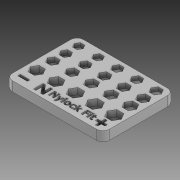
# Autodesk Inventor part: Standard Test Print
Saved by Autodesk Inventor 2022 (Build 260153000, 153)
## iProperties
Created: 2022-01-18
Part Number: Standard Test Print
Material: ABS Plastic
Document SubType Name: Modeling
Density: 1.06 g/cm^3
Appearance: Smooth - Medium Gray
Autodesk Inventor part; units mm, degrees
ref_plane "YZ Plane" through (0, 0, 0) normal (1, 0, 0) x (0, 1, 0)
ref_plane "XZ Plane" through (0, 0, 0) normal (0, 1, 0) x (-1, 0, 0)
ref_plane "XY Plane" through (0, 0, 0) normal (0, 0, 1) x (1, 0, 0)
sketch "Sketch1" plane through (0, 0, 0) normal (0, 1, 0) x (-1, 0, 0)
  line L0 (42.8625, 28.1781) -> (33.3375, 28.1781)
  line L1 (33.3375, 28.1781) -> (33.3375, 25.7969)
  line L2 (33.3375, 25.7969) -> (42.8625, 25.7969)
  line L3 (42.8625, 25.7969) -> (42.8625, 28.1781)
  line L4 (42.8625, 28.1781) -> (33.3375, 25.7969) construction
  line L5 (33.3375, 28.1781) -> (42.8625, 25.7969) construction
  line L6 (-33.3375, 28.1781) -> (-42.8625, 28.1781)
  line L7 (-42.8625, 28.1781) -> (-42.8625, 25.7969)
  line L8 (-42.8625, 25.7969) -> (-33.3375, 25.7969)
  line L9 (-33.3375, 25.7969) -> (-33.3375, 28.1781)
  line L10 (-33.3375, 28.1781) -> (-42.8625, 25.7969) construction
  line L11 (-42.8625, 28.1781) -> (-33.3375, 25.7969) construction
  line L12 (23.8125, 31.75) -> (23.8125, 22.225)
  line L13 (23.8125, 22.225) -> (21.4312, 22.225)
  line L14 (21.4312, 22.225) -> (16.6687, 28.0052)
  line L15 (16.6687, 28.0052) -> (16.6687, 22.225)
  line L16 (16.6687, 22.225) -> (14.2875, 22.225)
  line L17 (14.2875, 22.225) -> (14.2875, 31.75)
  line L18 (14.2875, 31.75) -> (16.6687, 31.75)
  line L19 (16.6687, 31.75) -> (21.4312, 25.9698)
  line L20 (21.4312, 25.9698) -> (21.4312, 31.75)
  line L21 (21.4312, 31.75) -> (23.8125, 31.75)
  line L22 (19.05, 28.8599) -> (19.05, 25.1151) construction
  line L23 (47.625, -34.925) -> (-47.625, -34.925)
  line L24 (-47.625, -34.925) -> (-47.625, 34.925)
  line L25 (-47.625, 34.925) -> (47.625, 34.925)
  line L26 (47.625, 34.925) -> (47.625, -34.925)
  line L27 (47.625, -34.925) -> (-47.625, 34.925) construction
  line L28 (-47.625, -34.925) -> (47.625, 34.925) construction
  line L29 (-39.2906, 22.225) -> (-36.9094, 22.225)
  line L30 (-36.9094, 22.225) -> (-36.9094, 31.75)
  line L31 (-36.9094, 31.75) -> (-39.2906, 31.75)
  line L32 (-39.2906, 31.75) -> (-39.2906, 22.225)
  line L33 (-39.2906, 22.225) -> (-36.9094, 31.75) construction
  line L34 (-36.9094, 22.225) -> (-39.2906, 31.75) construction
  line L35 (35.8086, -30.9562) -> (33.5173, -26.9875) construction
  line L36 (33.5173, -26.9875) -> (35.8086, -23.0187) construction
  line L37 (35.8086, -23.0187) -> (40.3914, -23.0187) construction
  line L38 (40.3914, -23.0187) -> (42.6827, -26.9875) construction
  line L39 (42.6827, -26.9875) -> (40.3914, -30.9563) construction
  line L40 (40.3914, -30.9563) -> (35.8086, -30.9562) construction
  line L41 (35.5795, -18.6531) -> (33.059, -14.2875) construction
  line L42 (33.059, -14.2875) -> (35.5795, -9.9219) construction
  line L43 (35.5795, -9.9219) -> (40.6205, -9.9219) construction
  line L44 (40.6205, -9.9219) -> (43.141, -14.2875) construction
  line L45 (43.141, -14.2875) -> (40.6205, -18.6531) construction
  line L46 (40.6205, -18.6531) -> (35.5795, -18.6531) construction
  line L47 (35.3504, -6.35) -> (32.6007, -1.5875) construction
  line L48 (32.6007, -1.5875) -> (35.3504, 3.175) construction
  line L49 (35.3504, 3.175) -> (40.8496, 3.175) construction
  line L50 (40.8496, 3.175) -> (43.5993, -1.5875) construction
  line L51 (43.5993, -1.5875) -> (40.8496, -6.35) construction
  line L52 (40.8496, -6.35) -> (35.3504, -6.35) construction
  line L53 (34.8921, 8.7312) -> (31.6842, 14.2875) construction
  line L54 (31.6842, 14.2875) -> (34.8921, 19.8437) construction
  line L55 (34.8921, 19.8437) -> (41.3079, 19.8438) construction
  line L56 (41.3079, 19.8438) -> (44.5158, 14.2875) construction
  line L57 (44.5158, 14.2875) -> (41.3079, 8.7312) construction
  line L58 (41.3079, 8.7312) -> (34.8921, 8.7312) construction
  line L59 (15.8421, 8.7312) -> (12.6342, 14.2875)
  line L60 (12.6342, 14.2875) -> (15.8421, 19.8437)
  line L61 (22.2579, 8.7312) -> (15.8421, 8.7312)
  line L62 (15.8421, 19.8437) -> (22.2579, 19.8438)
  line L63 (25.4658, 14.2875) -> (22.2579, 8.7312)
  line L64 (22.2579, 19.8438) -> (25.4658, 14.2875)
  line L65 (16.3004, 3.175) -> (21.7996, 3.175)
  line L66 (21.7996, 3.175) -> (24.5493, -1.5875)
  line L67 (24.5493, -1.5875) -> (21.7996, -6.35)
  line L68 (21.7996, -6.35) -> (16.3004, -6.35)
  line L69 (21.5705, -9.9219) -> (24.091, -14.2875)
  line L70 (16.5295, -18.6531) -> (14.009, -14.2875)
  line L71 (24.091, -14.2875) -> (21.5705, -18.6531)
  line L72 (21.5705, -18.6531) -> (16.5295, -18.6531)
  line L73 (16.7586, -23.0187) -> (21.3414, -23.0187)
  line L74 (14.4673, -26.9875) -> (16.7586, -23.0187)
  line L75 (16.7586, -30.9562) -> (14.4673, -26.9875)
  line L76 (21.3414, -30.9563) -> (16.7586, -30.9562)
  line L77 (21.3414, -23.0187) -> (23.6327, -26.9875)
  line L78 (23.6327, -26.9875) -> (21.3414, -30.9563)
  line L79 (16.5295, -9.9219) -> (21.5705, -9.9219)
  line L80 (13.5507, -1.5875) -> (16.3004, 3.175)
  line L81 (16.3004, -6.35) -> (13.5507, -1.5875)
  line L82 (14.009, -14.2875) -> (16.5295, -9.9219)
  line L83 (-3.2079, 8.7312) -> (-6.4158, 14.2875) construction
  line L84 (-6.4158, 14.2875) -> (-3.2079, 19.8437) construction
  line L85 (3.2079, 8.7312) -> (-3.2079, 8.7312) construction
  line L86 (-3.2079, 19.8437) -> (3.2079, 19.8438) construction
  line L87 (6.4158, 14.2875) -> (3.2079, 8.7312) construction
  line L88 (3.2079, 19.8438) -> (6.4158, 14.2875) construction
  line L89 (-2.7496, 3.175) -> (2.7496, 3.175) construction
  line L90 (2.7496, 3.175) -> (5.4993, -1.5875) construction
  line L91 (5.4993, -1.5875) -> (2.7496, -6.35) construction
  line L92 (2.7496, -6.35) -> (-2.7496, -6.35) construction
  line L93 (2.5205, -9.9219) -> (5.041, -14.2875) construction
  line L94 (-2.5205, -18.6531) -> (-5.041, -14.2875) construction
  line L95 (5.041, -14.2875) -> (2.5205, -18.6531) construction
  line L96 (2.5205, -18.6531) -> (-2.5205, -18.6531) construction
  line L97 (-2.2914, -23.0187) -> (2.2914, -23.0187) construction
  line L98 (-4.5827, -26.9875) -> (-2.2914, -23.0187) construction
  line L99 (-2.2914, -30.9562) -> (-4.5827, -26.9875) construction
  line L100 (2.2914, -30.9563) -> (-2.2914, -30.9562) construction
  line L101 (2.2914, -23.0187) -> (4.5827, -26.9875) construction
  line L102 (4.5827, -26.9875) -> (2.2914, -30.9563) construction
  line L103 (-2.5205, -9.9219) -> (2.5205, -9.9219) construction
  line L104 (-5.4993, -1.5875) -> (-2.7496, 3.175) construction
  line L105 (-2.7496, -6.35) -> (-5.4993, -1.5875) construction
  line L106 (-5.041, -14.2875) -> (-2.5205, -9.9219) construction
  line L107 (-22.2579, 8.7312) -> (-25.4658, 14.2875) construction
  line L108 (-25.4658, 14.2875) -> (-22.2579, 19.8437) construction
  line L109 (-15.8421, 8.7312) -> (-22.2579, 8.7312) construction
  line L110 (-22.2579, 19.8437) -> (-15.8421, 19.8438) construction
  line L111 (-12.6342, 14.2875) -> (-15.8421, 8.7312) construction
  line L112 (-15.8421, 19.8438) -> (-12.6342, 14.2875) construction
  line L113 (-21.7996, 3.175) -> (-16.3004, 3.175) construction
  line L114 (-16.3004, 3.175) -> (-13.5507, -1.5875) construction
  line L115 (-13.5507, -1.5875) -> (-16.3004, -6.35) construction
  line L116 (-16.3004, -6.35) -> (-21.7996, -6.35) construction
  line L117 (-16.5295, -9.9219) -> (-14.009, -14.2875) construction
  line L118 (-21.5705, -18.6531) -> (-24.091, -14.2875) construction
  line L119 (-14.009, -14.2875) -> (-16.5295, -18.6531) construction
  line L120 (-16.5295, -18.6531) -> (-21.5705, -18.6531) construction
  line L121 (-21.3414, -23.0187) -> (-16.7586, -23.0187) construction
  line L122 (-23.6327, -26.9875) -> (-21.3414, -23.0187) construction
  line L123 (-21.3414, -30.9562) -> (-23.6327, -26.9875) construction
  line L124 (-16.7586, -30.9563) -> (-21.3414, -30.9562) construction
  line L125 (-16.7586, -23.0187) -> (-14.4673, -26.9875) construction
  line L126 (-14.4673, -26.9875) -> (-16.7586, -30.9563) construction
  line L127 (-21.5705, -9.9219) -> (-16.5295, -9.9219) construction
  line L128 (-24.5493, -1.5875) -> (-21.7996, 3.175) construction
  line L129 (-21.7996, -6.35) -> (-24.5493, -1.5875) construction
  line L130 (-24.091, -14.2875) -> (-21.5705, -9.9219) construction
  line L131 (-41.3079, 8.7312) -> (-44.5158, 14.2875) construction
  line L132 (-44.5158, 14.2875) -> (-41.3079, 19.8437) construction
  line L133 (-34.8921, 8.7312) -> (-41.3079, 8.7312) construction
  line L134 (-41.3079, 19.8437) -> (-34.8921, 19.8438) construction
  line L135 (-31.6842, 14.2875) -> (-34.8921, 8.7312) construction
  line L136 (-34.8921, 19.8438) -> (-31.6842, 14.2875) construction
  line L137 (-40.8496, 3.175) -> (-35.3504, 3.175) construction
  line L138 (-35.3504, 3.175) -> (-32.6007, -1.5875) construction
  line L139 (-32.6007, -1.5875) -> (-35.3504, -6.35) construction
  line L140 (-35.3504, -6.35) -> (-40.8496, -6.35) construction
  line L141 (-35.5795, -9.9219) -> (-33.059, -14.2875) construction
  line L142 (-40.6205, -18.6531) -> (-43.141, -14.2875) construction
  line L143 (-33.059, -14.2875) -> (-35.5795, -18.6531) construction
  line L144 (-35.5795, -18.6531) -> (-40.6205, -18.6531) construction
  line L145 (-40.3914, -23.0187) -> (-35.8086, -23.0187) construction
  line L146 (-42.6827, -26.9875) -> (-40.3914, -23.0187) construction
  line L147 (-40.3914, -30.9562) -> (-42.6827, -26.9875) construction
  line L148 (-35.8086, -30.9563) -> (-40.3914, -30.9562) construction
  line L149 (-35.8086, -23.0187) -> (-33.5173, -26.9875) construction
  line L150 (-33.5173, -26.9875) -> (-35.8086, -30.9563) construction
  line L151 (-40.6205, -9.9219) -> (-35.5795, -9.9219) construction
  line L152 (-43.5993, -1.5875) -> (-40.8496, 3.175) construction
  line L153 (-40.8496, -6.35) -> (-43.5993, -1.5875) construction
  line L154 (-43.141, -14.2875) -> (-40.6205, -9.9219) construction
  line L155 (33.6639, -26.9875) -> (35.882, -30.8293)
  line L156 (35.882, -30.8293) -> (40.318, -30.8292)
  line L157 (40.318, -30.8292) -> (42.5361, -26.9875)
  line L158 (42.5361, -26.9875) -> (40.318, -23.1457)
  line L159 (40.318, -23.1457) -> (35.882, -23.1458)
  line L160 (35.882, -23.1458) -> (33.6639, -26.9875)
  line L161 (35.6528, -18.5261) -> (33.2057, -14.2875)
  line L162 (33.2057, -14.2875) -> (35.6528, -10.0489)
  line L163 (35.6528, -10.0489) -> (40.5472, -10.0489)
  line L164 (40.5472, -10.0489) -> (42.9943, -14.2875)
  line L165 (42.9943, -14.2875) -> (40.5472, -18.5261)
  line L166 (40.5472, -18.5261) -> (35.6528, -18.5261)
  line L167 (35.4237, -6.223) -> (32.7474, -1.5875)
  line L168 (32.7474, -1.5875) -> (35.4237, 3.048)
  line L169 (35.4237, 3.048) -> (40.7763, 3.048)
  line L170 (40.7763, 3.048) -> (43.4526, -1.5875)
  line L171 (43.4526, -1.5875) -> (40.7763, -6.223)
  line L172 (40.7763, -6.223) -> (35.4237, -6.223)
  line L173 (34.9654, 8.8583) -> (31.8308, 14.2875)
  line L174 (31.8308, 14.2875) -> (34.9654, 19.7167)
  line L175 (34.9654, 19.7167) -> (41.2346, 19.7167)
  line L176 (41.2346, 19.7167) -> (44.3692, 14.2875)
  line L177 (44.3692, 14.2875) -> (41.2346, 8.8583)
  line L178 (41.2346, 8.8583) -> (34.9654, 8.8583)
  line L179 (4.876, -26.9875) -> (2.438, -22.7647)
  line L180 (2.438, -22.7647) -> (-2.438, -22.7647)
  line L181 (-2.438, -22.7647) -> (-4.876, -26.9875)
  line L182 (-4.876, -26.9875) -> (-2.438, -31.2102)
  line L183 (-2.438, -31.2102) -> (2.438, -31.2102)
  line L184 (2.438, -31.2102) -> (4.876, -26.9875)
  line L185 (2.6671, -18.9071) -> (5.3343, -14.2875)
  line L186 (5.3343, -14.2875) -> (2.6671, -9.6679)
  line L187 (2.6671, -9.6679) -> (-2.6671, -9.6679)
  line L188 (-2.6671, -9.6679) -> (-5.3343, -14.2875)
  line L189 (-5.3343, -14.2875) -> (-2.6671, -18.9071)
  line L190 (-2.6671, -18.9071) -> (2.6671, -18.9071)
  line L191 (5.7926, -1.5875) -> (2.8963, 3.429)
  line L192 (2.8963, 3.429) -> (-2.8963, 3.429)
  line L193 (-2.8963, 3.429) -> (-5.7926, -1.5875)
  line L194 (-5.7926, -1.5875) -> (-2.8963, -6.604)
  line L195 (-2.8963, -6.604) -> (2.8963, -6.604)
  line L196 (2.8963, -6.604) -> (5.7926, -1.5875)
  line L197 (3.3545, 8.4773) -> (6.7091, 14.2875)
  line L198 (6.7091, 14.2875) -> (3.3545, 20.0977)
  line L199 (3.3545, 20.0977) -> (-3.3545, 20.0977)
  line L200 (-3.3545, 20.0977) -> (-6.7091, 14.2875)
  line L201 (-6.7091, 14.2875) -> (-3.3545, 8.4773)
  line L202 (-3.3545, 8.4773) -> (3.3545, 8.4773)
  line L203 (-12.1943, 14.2875) -> (-15.6221, 20.2247)
  line L204 (-15.6221, 20.2247) -> (-22.4779, 20.2247)
  line L205 (-22.4779, 20.2247) -> (-25.9057, 14.2875)
  line L206 (-25.9057, 14.2875) -> (-22.4779, 8.3502)
  line L207 (-22.4779, 8.3502) -> (-15.6221, 8.3502)
  line L208 (-15.6221, 8.3502) -> (-12.1943, 14.2875)
  line L209 (-13.1108, -1.5875) -> (-16.0804, 3.556)
  line L210 (-16.0804, 3.556) -> (-22.0196, 3.556)
  line L211 (-22.0196, 3.556) -> (-24.9892, -1.5875)
  line L212 (-24.9892, -1.5875) -> (-22.0196, -6.731)
  line L213 (-22.0196, -6.731) -> (-16.0804, -6.731)
  line L214 (-16.0804, -6.731) -> (-13.1108, -1.5875)
  line L215 (-13.5691, -14.2875) -> (-16.3095, -9.5409)
  line L216 (-16.3095, -9.5409) -> (-21.7905, -9.5409)
  line L217 (-21.7905, -9.5409) -> (-24.5309, -14.2875)
  line L218 (-24.5309, -14.2875) -> (-21.7905, -19.0341)
  line L219 (-21.7905, -19.0341) -> (-16.3095, -19.0341)
  line L220 (-16.3095, -19.0341) -> (-13.5691, -14.2875)
  line L221 (-14.0273, -26.9875) -> (-16.5387, -22.6378)
  line L222 (-16.5387, -22.6378) -> (-21.5613, -22.6378)
  line L223 (-21.5613, -22.6378) -> (-24.0727, -26.9875)
  line L224 (-24.0727, -26.9875) -> (-21.5613, -31.3372)
  line L225 (-21.5613, -31.3372) -> (-16.5387, -31.3372)
  line L226 (-16.5387, -31.3372) -> (-14.0273, -26.9875)
  line L227 (-35.5153, -31.4642) -> (-32.9307, -26.9875)
  line L228 (-32.9307, -26.9875) -> (-35.5153, -22.5108)
  line L229 (-35.5153, -22.5108) -> (-40.6847, -22.5108)
  line L230 (-40.6847, -22.5108) -> (-43.2693, -26.9875)
  line L231 (-43.2693, -26.9875) -> (-40.6847, -31.4642)
  line L232 (-40.6847, -31.4642) -> (-35.5153, -31.4642)
  line L233 (-32.4724, -14.2875) -> (-35.2862, -9.4139)
  line L234 (-35.2862, -9.4139) -> (-40.9138, -9.4139)
  line L235 (-40.9138, -9.4139) -> (-43.7276, -14.2875)
  line L236 (-43.7276, -14.2875) -> (-40.9138, -19.1611)
  line L237 (-40.9138, -19.1611) -> (-35.2862, -19.1611)
  line L238 (-35.2862, -19.1611) -> (-32.4724, -14.2875)
  line L239 (-32.0142, -1.5875) -> (-35.0571, 3.683)
  line L240 (-35.0571, 3.683) -> (-41.1429, 3.683)
  line L241 (-41.1429, 3.683) -> (-44.1858, -1.5875)
  line L242 (-44.1858, -1.5875) -> (-41.1429, -6.858)
  line L243 (-41.1429, -6.858) -> (-35.0571, -6.858)
  line L244 (-35.0571, -6.858) -> (-32.0142, -1.5875)
  line L245 (-34.5988, 8.2233) -> (-31.0976, 14.2875)
  line L246 (-31.0976, 14.2875) -> (-34.5988, 20.3518)
  line L247 (-34.5988, 20.3518) -> (-41.6012, 20.3518)
  line L248 (-41.6012, 20.3518) -> (-45.1024, 14.2875)
  line L249 (-45.1024, 14.2875) -> (-41.6012, 8.2233)
  line L250 (-41.6012, 8.2233) -> (-34.5988, 8.2233)
  line L251 (16.0071, 23.8369) -> (-35.0571, 23.8369) construction
  line L252 (-35.0571, 23.8369) -> (-35.0571, 30.1381) construction
  line L253 (-35.0571, 30.1381) -> (16.0071, 30.1381) construction
  line L254 (16.0071, 30.1381) -> (16.0071, 23.8369) construction
  line L255 (6.1493, 29.4292) -> (7.6828, 29.4292)
  line L256 (7.6828, 29.4292) -> (10.1322, 25.0038)
  line L257 (10.1322, 25.0038) -> (10.1322, 29.4292)
  line L258 (10.1322, 29.4292) -> (11.5885, 29.4292)
  line L259 (11.5885, 29.4292) -> (11.5885, 23.0792)
  line L260 (11.5885, 23.0792) -> (9.6331, 23.0792)
  line L261 (9.6331, 23.0792) -> (7.6056, 26.7173)
  line L262 (7.6056, 26.7173) -> (7.6056, 23.0792)
  line L263 (7.6056, 23.0792) -> (6.1493, 23.0792)
  line L264 (6.1493, 23.0792) -> (6.1493, 29.4292)
  line L265 (0.4786, 24.6384) -> (2.892, 31.184)
  line L266 (2.892, 31.184) -> (4.4975, 31.184)
  line L267 (4.4975, 31.184) -> (3.7719, 29.3109)
  line L268 (3.7719, 29.3109) -> (5.5267, 24.6384)
  line L269 (5.5267, 24.6384) -> (3.9623, 24.6384)
  line L270 (3.9623, 24.6384) -> (2.9537, 27.6436)
  line L271 (2.9537, 27.6436) -> (2.012, 24.6384)
  line L272 (2.012, 24.6384) -> (0.4786, 24.6384)
  line L273 (-1.5746, 29.4292) -> (-0.0823, 29.4292)
  line L274 (-0.0823, 29.4292) -> (-0.0823, 22.7962)
  line L275 (-0.0823, 22.7962) -> (-1.5746, 22.7962)
  line L276 (-1.5746, 22.7962) -> (-1.5746, 29.4292)
  spline S0 degree 2 poles (-7.3123, 27.0364) (-7.3123, 28.2199) (-6.0207, 29.5784) (-4.8423, 29.5784) knots 0 0 0 1 2 2 2
  spline S1 degree 2 poles (-4.8423, 29.5784) (-3.669, 29.5784) (-2.3671, 28.2199) (-2.3671, 27.0364) knots 0 0 0 1 2 2 2
  spline S2 degree 2 poles (-2.3671, 27.0364) (-2.3671, 25.8425) (-3.669, 24.4892) (-4.8423, 24.4892) knots 0 0 0 1 2 2 2
  spline S3 degree 2 poles (-4.8423, 24.4892) (-6.0155, 24.4892) (-7.3123, 25.8477) (-7.3123, 27.0364) knots 0 0 0 1 2 2 2
  spline S4 degree 2 poles (-5.784, 27.0467) (-5.784, 26.6196) (-5.645, 26.0484) (-5.5215, 25.8786) knots 0 0 0 1 2 2 2
  spline S5 degree 2 poles (-5.5215, 25.8786) (-5.3877, 25.6985) (-5.0532, 25.5595) (-4.8423, 25.5595) knots 0 0 0 1 2 2 2
  spline S6 degree 2 poles (-4.8423, 25.5595) (-4.6364, 25.5595) (-4.3122, 25.683) (-4.1784, 25.858) knots 0 0 0 1 2 2 2
  spline S7 degree 2 poles (-4.1784, 25.858) (-4.0498, 26.0226) (-3.8954, 26.6041) (-3.8954, 27.0467) knots 0 0 0 1 2 2 2
  spline S8 degree 2 poles (-3.8954, 27.0467) (-3.8954, 27.4841) (-4.0395, 28.0244) (-4.1579, 28.1891) knots 0 0 0 1 2 2 2
  spline S9 degree 2 poles (-4.1579, 28.1891) (-4.2762, 28.3537) (-4.6364, 28.5081) (-4.8526, 28.5081) knots 0 0 0 1 2 2 2
  spline S10 degree 2 poles (-4.8526, 28.5081) (-5.0327, 28.5081) (-5.4032, 28.3537) (-5.5164, 28.1994) knots 0 0 0 1 2 2 2
  spline S11 degree 2 poles (-5.5164, 28.1994) (-5.645, 28.0192) (-5.784, 27.4995) (-5.784, 27.0467) knots 0 0 0 1 2 2 2
  spline S12 degree 2 poles (-10.4513, 29.5579) (-9.8595, 29.5579) (-8.8766, 29.2594) (-8.5113, 28.9506) knots 0 0 0 1 2 2 2
  spline S13 degree 2 poles (-8.5113, 28.9506) (-8.1562, 28.6368) (-7.7548, 27.6951) (-7.7548, 27.057) knots 0 0 0 1 2 2 2
  spline S14 degree 2 poles (-7.7548, 27.057) (-7.7548, 26.3674) (-8.1871, 25.4051) (-8.5627, 25.0964) knots 0 0 0 1 2 2 2
  spline S15 degree 2 poles (-8.5627, 25.0964) (-8.9178, 24.7979) (-9.8852, 24.5098) (-10.4101, 24.5098) knots 0 0 0 1 2 2 2
  spline S16 degree 2 poles (-10.4101, 24.5098) (-10.8063, 24.5098) (-11.5988, 24.695) (-12.0002, 24.8957) knots 0 0 0 1 2 2 2
  line L277 (-12.0002, 24.8957) -> (-12.0002, 26.1719)
  line L278 (-12.0002, 26.1719) -> (-11.8098, 26.1719)
  spline S17 degree 2 poles (-11.8098, 26.1719) (-11.7171, 26.0844) (-11.4598, 25.8786) (-11.3055, 25.7962) knots 0 0 0 1 2 2 2
  spline S18 degree 2 poles (-11.3055, 25.7962) (-11.1408, 25.7036) (-10.7343, 25.5801) (-10.4821, 25.5801) knots 0 0 0 1 2 2 2
  spline S19 degree 2 poles (-10.4821, 25.5801) (-9.9109, 25.5801) (-9.2831, 26.3777) (-9.2831, 27.057) knots 0 0 0 1 2 2 2
  spline S20 degree 2 poles (-9.2831, 27.057) (-9.2831, 27.7774) (-9.9521, 28.4875) (-10.5079, 28.4875) knots 0 0 0 1 2 2 2
  spline S21 degree 2 poles (-10.5079, 28.4875) (-10.7909, 28.4875) (-11.2128, 28.3589) (-11.3672, 28.2662) knots 0 0 0 1 2 2 2
  spline S22 degree 2 poles (-11.3672, 28.2662) (-11.5165, 28.1788) (-11.7326, 27.9832) (-11.8098, 27.906) knots 0 0 0 1 2 2 2
  line L279 (-11.8098, 27.906) -> (-12.0002, 27.906)
  line L280 (-12.0002, 27.906) -> (-12.0002, 29.1874)
  spline S23 degree 2 poles (-12.0002, 29.1874) (-11.8715, 29.244) (-11.537, 29.388) (-11.3621, 29.4344) knots 0 0 0 1 2 2 2
  spline S24 degree 2 poles (-11.3621, 29.4344) (-11.1459, 29.4961) (-10.7652, 29.5579) (-10.4513, 29.5579) knots 0 0 0 1 2 2 2
  line L281 (-17.5062, 29.4292) -> (-15.7309, 29.4292)
  line L282 (-15.7309, 29.4292) -> (-14.4342, 27.3503)
  line L283 (-14.4342, 27.3503) -> (-14.2026, 27.659)
  line L284 (-14.2026, 27.659) -> (-14.2026, 29.4292)
  line L285 (-14.2026, 29.4292) -> (-12.7103, 29.4292)
  line L286 (-12.7103, 29.4292) -> (-12.7103, 22.7962)
  line L287 (-12.7103, 22.7962) -> (-14.2026, 22.7962)
  line L288 (-14.2026, 22.7962) -> (-14.2026, 26.5115)
  line L289 (-14.2026, 26.5115) -> (-15.6177, 24.6384)
  line L290 (-15.6177, 24.6384) -> (-17.3827, 24.6384)
  line L291 (-17.3827, 24.6384) -> (-15.7052, 26.7019)
  line L292 (-15.7052, 26.7019) -> (-17.5062, 29.4292)
  line L293 (-24.87, 24.2885) -> (-22.2044, 24.2885)
  line L294 (-22.2044, 24.2885) -> (-22.2044, 25.4875)
  line L295 (-22.2044, 25.4875) -> (-24.659, 25.4875)
  line L296 (-24.659, 25.4875) -> (-24.659, 26.6968)
  line L297 (-24.659, 26.6968) -> (-22.2044, 26.6968)
  line L298 (-22.2044, 26.6968) -> (-22.2044, 29.4292)
  line L299 (-22.2044, 29.4292) -> (-20.6195, 29.4292)
  line L300 (-20.6195, 29.4292) -> (-20.6195, 23.0792)
  line L301 (-20.6195, 23.0792) -> (-24.87, 23.0792)
  line L302 (-24.87, 23.0792) -> (-24.87, 24.2885)
  line L303 (-27.0981, 29.4292) -> (-25.6058, 29.4292)
  line L304 (-25.6058, 29.4292) -> (-25.6058, 24.6384)
  line L305 (-25.6058, 24.6384) -> (-27.0981, 24.6384)
  line L306 (-27.0981, 24.6384) -> (-27.0981, 29.4292)
  line L307 (-27.1444, 23.954) -> (-25.5647, 23.954)
  line L308 (-25.5647, 23.954) -> (-25.5647, 22.791)
  line L309 (-25.5647, 22.791) -> (-27.1444, 22.791)
  line L310 (-27.1444, 22.791) -> (-27.1444, 23.954)
  spline S25 degree 2 poles (-30.0724, 29.5218) (-29.1616, 29.5218) (-28.328, 28.7705) (-28.328, 27.9163) knots 0 0 0 1 2 2 2
  line L311 (-28.328, 27.9163) -> (-28.328, 25.6779)
  line L312 (-28.328, 25.6779) -> (-27.7568, 25.6779)
  line L313 (-27.7568, 25.6779) -> (-27.7568, 24.6384)
  line L314 (-27.7568, 24.6384) -> (-28.328, 24.6384)
  line L315 (-28.328, 24.6384) -> (-28.328, 23.2696)
  line L316 (-28.328, 23.2696) -> (-29.8203, 23.2696)
  line L317 (-29.8203, 23.2696) -> (-29.8203, 24.6384)
  line L318 (-29.8203, 24.6384) -> (-31.2611, 24.6384)
  line L319 (-31.2611, 24.6384) -> (-31.2611, 25.6779)
  line L320 (-31.2611, 25.6779) -> (-29.8203, 25.6779)
  line L321 (-29.8203, 25.6779) -> (-29.8203, 27.3812)
  spline S26 degree 2 poles (-29.8203, 27.3812) (-29.8203, 27.6333) (-29.8306, 28.009) (-29.8923, 28.1582) knots 0 0 0 1 2 2 2
  spline S27 degree 2 poles (-29.8923, 28.1582) (-29.9541, 28.3074) (-30.2577, 28.4824) (-30.5459, 28.4824) knots 0 0 0 1 2 2 2
  spline S28 degree 2 poles (-30.5459, 28.4824) (-30.6694, 28.4824) (-31.0553, 28.3795) (-31.1325, 28.3383) knots 0 0 0 1 2 2 2
  line L322 (-31.1325, 28.3383) -> (-31.2611, 28.3383)
  line L323 (-31.2611, 28.3383) -> (-31.2611, 29.388)
  spline S29 degree 2 poles (-31.2611, 29.388) (-31.0193, 29.4498) (-30.4738, 29.5218) (-30.0724, 29.5218) knots 0 0 0 1 2 2 2
  point P0 (38.1, 26.9875)
  point P1 (-38.1, 26.9875)
  point P2 (-38.1, 26.9875)
  point P3 (38.1, 26.9875)
  point P4 (-38.1, 26.9875)
  point P5 (38.1, 26.9875)
  point P6 (19.05, 26.9875)
  point P7 (-39.2906, 28.1781)
  point P8 (-36.9094, 28.1781)
  point P9 (-36.9094, 25.7969)
  point P10 (-39.2906, 25.7969)
  point P11 (38.1, -26.9875)
  point P12 (38.1, -14.2875)
  point P13 (38.1, -1.5875)
  point P14 (38.1, 14.2875)
  point P15 (0, 0)
  point P16 (19.05, 14.2875)
  point P17 (19.05, -26.9875)
  point P18 (19.05, -14.2875)
  point P19 (19.05, -1.5875)
  point P20 (0, 14.2875)
  point P21 (0, -26.9875)
  point P22 (0, -14.2875)
  point P23 (0, -1.5875)
  point P24 (-19.05, 14.2875)
  point P25 (-19.05, -26.9875)
  point P26 (-19.05, -14.2875)
  point P27 (-19.05, -1.5875)
  point P28 (-38.1, 14.2875)
  point P29 (-38.1, -26.9875)
  point P30 (-38.1, -14.2875)
  point P31 (-38.1, -1.5875)
  point P32 (0, 0)
  point P33 (-38.1, 26.9875)
  point P34 (16.0071, 26.9875)
  point P35 (-9.525, 23.8369)
  dimension "d33" = 9.525
  dimension "d34" = 2.3813
  dimension "d61" = 9.525
  dimension "d62" = 9.525
  dimension "d64" = 2.3813
  dimension "d121" = 69.85
  dimension "d124" = 95.25
  dimension "d131" = 7.9375
  dimension "d132" = 8.7312
  dimension "d133" = 9.525
  dimension "d134" = 11.1125
  dimension "d135" = 15.875
  dimension "d136" = 12.7
  dimension "d137" = 12.7
  dimension "d138" = 12.7
  dimension "d139" = 53.975
  dimension "d140" = 26.9875
  dimension "d143" = 19.05
  dimension "d148" = 0.127
  dimension "d149" = 0.127
  dimension "d150" = 0.127
  dimension "d151" = 0.127
  dimension "d152" = 0.254
  dimension "d153" = 0.254
  dimension "d154" = 0.254
  dimension "d155" = 0.254
  dimension "d156" = 0.381
  dimension "d157" = 0.381
  dimension "d158" = 0.381
  dimension "d159" = 0.381
  dimension "d160" = 0.508
  dimension "d161" = 0.508
  dimension "d162" = 0.508
  dimension "d163" = 0.508
  dimension "d172" = 9.525
  constraints: 503 end point, 18 midpoint, 11 parallel, 9 horizontal, 7 equal length, 7 perpendicular, 7 vertical alignment, 6 point on line, 3 horizontal alignment, 2 vertical, 342 other
  measures "d33" distance of L1.end L2.end
  measures "d34" distance of L2.end L0.start
  measures "d61" distance between parallel lines of L17 L12
  measures "d62" distance between parallel lines of L18 L16
  measures "d64" distance between parallel lines of L19 L14
  measures "d121" distance of L25.end L23.start
  measures "d124" distance of L23.start L23.end
  measures "d131" distance between parallel lines of L37 L40
  measures "d132" distance between parallel lines of L43 L46
  measures "d133" distance between parallel lines of L49 L52
  measures "d134" distance between parallel lines of L55 L58
  measures "d135" distance of point (38.1, -1.587) point (38.1, 14.287)
  measures "d136" distance of point (38.1, -14.287) point (38.1, -1.587)
  measures "d137" distance of point (38.1, -26.988) point (38.1, -14.287)
  measures "d138" distance of point (38.1, 14.287) point (38.1, 26.988)
  measures "d139" distance of point (38.1, 26.988) point (38.1, -26.988)
  measures "d140" vertical distance of point (0, 0) point (38.1, -26.988)
  measures "d143" distance of L53.start L59.start
  measures "d148" distance between parallel lines of L35 L155
  measures "d149" distance between parallel lines of L46 L166
  measures "d150" distance between parallel lines of L52 L172
  measures "d151" distance between parallel lines of L58 L178
  measures "d152" distance between parallel lines of L183 L100
  measures "d153" distance between parallel lines of L96 L190
  measures "d154" distance between parallel lines of L92 L195
  measures "d155" distance between parallel lines of L85 L202
  measures "d156" distance between parallel lines of L225 L124
  measures "d157" distance between parallel lines of L219 L120
  measures "d158" distance between parallel lines of L213 L116
  measures "d159" distance between parallel lines of L207 L109
  measures "d160" distance between parallel lines of L232 L148
  measures "d161" distance between parallel lines of L237 L144
  measures "d162" distance between parallel lines of L243 L140
  measures "d163" distance between parallel lines of L250 L133
  measures "d172" horizontal distance of point (-9.525, 23.837) point (0, 14.287)
extrude "Extrusion1" add sketch "Sketch1" against normal blind 9.525 contours L23 L24 L25 L26 | L59 L60 L62 L64 L63 L61 | L65 L66 L67 L68 L81 L80 | L69 L71 L72 L70 L82 L79 | L73 L77 L78 L76 L75 L74 | L160 L159 L158 L157 L156 L155 | L161 L162 L163 L164 L165 L166 | L167 L168 L169 L170 L171 L172 | L173 L174 L175 L176 L177 L178 | L184 L183 L182 L181 L180 L179 | L190 L189 L188 L187 L186 L185 | L196 L195 L194 L193 L192 L191 | L202 L201 L200 L199 L198 L197 | L208 L207 L206 L205 L204 L203 | L214 L213 L212 L211 L210 L209 | L220 L219 L218 L217 L216 L215 | L226 L225 L224 L223 L222 L221 | L232 L231 L230 L229 L228 L227 | L238 L237 L236 L235 L234 L233 | L244 L243 L242 L241 L240 L239 | L250 L249 L248 L247 L246 L245 | L255 L256 L257 L258 L259 L260 L261 L262 L263 L264 | L265 L266 L267 L268 L269 L270 L271 L272 | L273 L274 L275 L276 | S0 S1 S2 S3 | S11 S10 S9 S8 S7 S6 S5 S4 | S12 S13 S14 S15 S16 L277 L278 S17 S18 S19 S20 S21 S22 L279 L280 S23 S24 | L281 L282 L283 L284 L285 L286 L287 L288 L289 L290 L291 L292 | L293 L294 L295 L296 L297 L298 L299 L300 L301 L302 | L303 L304 L305 L306 | L307 L308 L309 L310 | S25 L311 L312 L313 L314 L315 L316 L317 L318 L319 L320 L321 S26 S27 S28 L322 L323 S29
fillet "Fillet1" radius 6.35 4 edges at (-47.625, -4.7625, 34.925) (-47.625, -4.7625, -34.925) (47.625, -4.7625, -34.925) (47.625, -4.7625, 34.925)
fillet "Fillet2" radius 0.3969 26 edges at (-16.6687, -4.7625, 28.0052) (42.8625, -4.7625, 25.7969) (42.8625, -4.7625, 28.1781) (33.3375, -4.7625, 28.1781) (33.3375, -4.7625, 25.7969) (-16.6687, -4.7625, 22.225) (-14.2875, -4.7625, 22.225) (-14.2875, -4.7625, 31.75) (-16.6687, -4.7625, 31.75) (-21.4312, -4.7625, 25.9698) (-21.4312, -4.7625, 22.225) (-23.8125, -4.7625, 22.225) (-21.4312, -4.7625, 31.75) (-23.8125, -4.7625, 31.75) (-33.3375, -4.7625, 28.1781) (-33.3375, -4.7625, 25.7969) (-42.8625, -4.7625, 25.7969) (-42.8625, -4.7625, 28.1781) (36.9094, -4.7625, 25.7969) (39.2906, -4.7625, 25.7969) (39.2906, -4.7625, 22.225) (36.9094, -4.7625, 22.225) (36.9094, -4.7625, 31.75) (36.9094, -4.7625, 28.1781) (39.2906, -4.7625, 31.75) (39.2906, -4.7625, 28.1781)
extrude "Extrusion2" cut sketch "Sketch1" against normal blind 3.81 contours L73 L77 L78 L76 L75 L74 | L160 L159 L158 L157 L156 L155 | L184 L183 L182 L181 L180 L179 | L226 L225 L224 L223 L222 L221 | L232 L231 L230 L229 L228 L227
extrude "Extrusion3" cut sketch "Sketch1" against normal blind 4.7625 contours L65 L66 L67 L68 L81 L80 | L69 L71 L72 L70 L82 L79 | L161 L162 L163 L164 L165 L166 | L167 L168 L169 L170 L171 L172 | L190 L189 L188 L187 L186 L185 | L196 L195 L194 L193 L192 L191 | L214 L213 L212 L211 L210 L209 | L220 L219 L218 L217 L216 L215 | L238 L237 L236 L235 L234 L233 | L244 L243 L242 L241 L240 L239
extrude "Extrusion4" cut sketch "Sketch1" against normal blind 6.35 contours L59 L60 L62 L64 L63 L61 | L173 L174 L175 L176 L177 L178 | L202 L201 L200 L199 L198 L197 | L208 L207 L206 L205 L204 L203 | L250 L249 L248 L247 L246 L245
emboss "Emboss1" sketch "Sketch1" operation cut depth 3.175 direction (0, -1, 0) contours L255 L256 L257 L258 L259 L260 L261 L262 L263 L264 | L265 L266 L267 L268 L269 L270 L271 L272 | L273 L274 L275 L276 | S0 S1 S2 S3 | S12 S13 S14 S15 S16 L277 L278 S17 S18 S19 S20 S21 S22 L279 L280 S23 S24 | L281 L282 L283 L284 L285 L286 L287 L288 L289 L290 L291 L292 | L293 L294 L295 L296 L297 L298 L299 L300 L301 L302 | L303 L304 L305 L306 | L307 L308 L309 L310 | S25 L311 L312 L313 L314 L315 L316 L317 L318 L319 L320 L321 S26 S27 S28 L322 L323 S29
body "Solid1"
